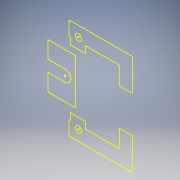
# Autodesk Inventor part: plate
Saved by Autodesk Inventor 2019 (Build 230136000, 136)
## iProperties
Created: 2019-10-25
Part Number: plate
Material: Generic
Document SubType Name: Modeling
Designer: marsikovabarbora
Density: 1 g/cm^3
Appearance: Default
Author: marsikovabarbora
Autodesk Inventor part; units mm, degrees
ref_plane "YZ Plane" through (0, 0, 0) normal (1, 0, 0) x (0, 1, 0)
ref_plane "XZ Plane" through (0, 0, 0) normal (0, 1, 0) x (-1, 0, 0)
ref_plane "XY Plane" through (0, 0, 0) normal (0, 0, 1) x (1, 0, 0)
sketch "Sketch1" plane through (0, 0, 0) normal (0, 0, 1) x (1, 0, 0)
  circle A0 centre (-17.8844, -9.45) radius 1.4 construction
  line L0 (-22, -13.95) -> (-22, -7.7794) construction
  line L1 (5.75, -13.95) -> (-22, -13.95) construction
  line L2 (5.75, 0) -> (5.75, -13.95) construction
  line L3 (5.75, 0) -> (0, 0) construction
  line L4 (0, 0) -> (0, -7.7794) construction
  line L5 (-14.8242, -7.7794) -> (0, -7.7794) construction
  line L6 (-14.8242, -4.7794) -> (-14.8242, -7.7794) construction
  line L7 (-21.3713, -4.7794) -> (-14.8242, -4.7794) construction
  line L8 (-21.3713, -7.7794) -> (-21.3713, -4.7794) construction
  line L9 (-22, -7.7794) -> (-21.3713, -7.7794) construction
  circle A1 centre (-17.8844, 25.55) radius 1.4 construction
  line L10 (-22, 23.8794) -> (-22, 30.05) construction
  line L11 (-22, 23.8794) -> (-21.3713, 23.8794) construction
  line L12 (-21.3713, 20.8794) -> (-21.3713, 23.8794) construction
  line L13 (-14.8242, 20.8794) -> (-21.3713, 20.8794) construction
  line L14 (-14.8242, 23.8794) -> (-14.8242, 20.8794) construction
  line L15 (-14.8242, 23.8794) -> (0, 23.8794) construction
  line L16 (0, 16.1) -> (0, 23.8794) construction
  line L17 (5.75, 16.1) -> (0, 16.1) construction
  line L18 (5.75, 16.1) -> (5.75, 30.05) construction
  line L19 (5.75, 30.05) -> (-22, 30.05) construction
  line L20 (-23.6597, 10.55) -> (-31.2138, 10.55) construction
  arc A2 (-23.6597, 5.55) -> (-23.6597, 10.55) centre (-23.6597, 8.05) ccw construction
  line L21 (-31.2138, 5.55) -> (-23.6597, 5.55) construction
  line L22 (-31.2138, 5.55) -> (-31.2138, -1.8612) construction
  line L23 (-19.2138, -1.8612) -> (-31.2138, -1.8612) construction
  line L24 (-19.2138, 17.9612) -> (-19.2138, -1.8612) construction
  line L25 (-31.2138, 17.9612) -> (-19.2138, 17.9612) construction
  line L26 (-31.2138, 17.9612) -> (-31.2138, 10.55) construction
  line L27 (5.75, 30.05) -> (-34.7444, 30.05)
  line L28 (-34.7444, 30.05) -> (-34.7444, -13.95)
  line L29 (-34.7444, -13.95) -> (5.75, -13.95)
  line L30 (5.75, -13.95) -> (5.75, 30.05)
  circle A3 centre (-17.8844, 25.55) radius 1.4
  circle A4 centre (-17.8844, -9.45) radius 1.4
  line L31 (-23.6597, 8.05) -> (-27.2138, 8.05) construction
  line L32 (-23.6597, 12.05) -> (-27.2138, 12.05)
  line L33 (-27.2138, 4.05) -> (-23.6597, 4.05)
  arc A5 (-23.6597, 4.05) -> (-23.6597, 12.05) centre (-23.6597, 8.05) ccw
  arc A6 (-27.2138, 12.05) -> (-27.2138, 4.05) centre (-27.2138, 8.05) ccw
  point P0 (-25.4367, 8.05)
  dimension "d2" = 8
  constraints: 16 end point, 5 tangent, 4 centre point, 4 point on circle, 3 parallel, 2 coincident, 2 concentric, 2 horizontal, 1 collinear, 1 midpoint, 1 perpendicular
  measures "d2" diameter of A6
extrude "Extrusion1" add sketch "Sketch1" along normal blind 5.5
body "Solid1"
